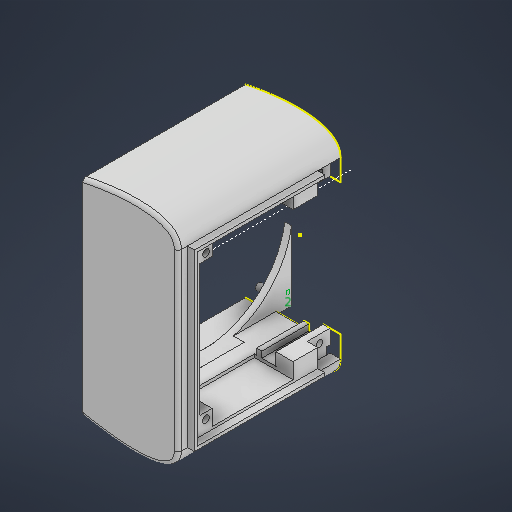
# Autodesk Inventor part: BP_FrontHSCover
Saved by Autodesk Inventor 2026.1 (Build 301233020, 233B)
## iProperties
Created: 2025-09-12
Part Number: BP_FrontHSCover
Material: Generic
Document SubType Name: Modeling
Designer: atrus
Density: 1 g/cm^3
Appearance: Default
Author: atrus
Autodesk Inventor part; units mm, degrees
ref_plane "YZ Plane" through (0, 0, 0) normal (1, 0, 0) x (0, 1, 0)
ref_plane "XZ Plane" through (0, 0, 0) normal (0, 1, 0) x (-1, 0, 0)
ref_plane "XY Plane" through (0, 0, 0) normal (0, 0, 1) x (1, 0, 0)
ref_plane "Work Plane1" through (0, 0, 0) normal (0, 0, 1) x (1, 0, 0)
sketch "Sketch1" plane through (0, 0, 0) normal (0, 0, 1) x (1, 0, 0)
  line L0 (13.335, 44.45) -> (13.335, -44.45) construction
  line L1 (5.715, 44.45) -> (13.335, 44.45) construction
  line L2 (5.715, 40.1825) -> (5.715, 44.45) construction
  arc A0 (4.9739, 39.4208) -> (5.715, 40.1825) centre (4.953, 40.1825) ccw construction
  line L3 (-12.5939, 38.9379) -> (4.9739, 39.4208) construction
  arc A1 (-12.5939, 38.9379) -> (-12.5939, 37.4145) centre (-12.573, 38.1762) ccw construction
  line L4 (4.9739, 36.9316) -> (-12.5939, 37.4145) construction
  arc A2 (5.715, 36.1699) -> (4.9739, 36.9316) centre (4.953, 36.1699) ccw construction
  line L5 (5.715, 29.2859) -> (5.715, 36.1699) construction
  arc A3 (4.9739, 28.5242) -> (5.715, 29.2859) centre (4.953, 29.2859) ccw construction
  line L6 (-12.5939, 28.0413) -> (4.9739, 28.5242) construction
  arc A4 (-12.5939, 28.0413) -> (-12.5939, 26.5179) centre (-12.573, 27.2796) ccw construction
  line L7 (4.9739, 26.035) -> (-12.5939, 26.5179) construction
  arc A5 (5.715, 25.2733) -> (4.9739, 26.035) centre (4.953, 25.2733) ccw construction
  line L8 (5.715, 18.3893) -> (5.715, 25.2733) construction
  arc A6 (4.9739, 17.6276) -> (5.715, 18.3893) centre (4.953, 18.3893) ccw construction
  line L9 (-12.5939, 17.1447) -> (4.9739, 17.6276) construction
  arc A7 (-12.5939, 17.1447) -> (-12.5939, 15.6213) centre (-12.573, 16.383) ccw construction
  line L10 (4.9739, 15.1384) -> (-12.5939, 15.6213) construction
  arc A8 (5.715, 14.3767) -> (4.9739, 15.1384) centre (4.953, 14.3767) ccw construction
  line L11 (5.715, 7.4927) -> (5.715, 14.3767) construction
  arc A9 (4.9739, 6.731) -> (5.715, 7.4927) centre (4.953, 7.4927) ccw construction
  line L12 (-12.5939, 6.2481) -> (4.9739, 6.731) construction
  arc A10 (-12.5939, 6.2481) -> (-12.5939, 4.7247) centre (-12.573, 5.4864) ccw construction
  line L13 (4.9739, 4.2418) -> (-12.5939, 4.7247) construction
  arc A11 (5.715, 3.4801) -> (4.9739, 4.2418) centre (4.953, 3.4801) ccw construction
  line L14 (5.715, -3.4039) -> (5.715, 3.4801) construction
  arc A12 (4.9739, -4.1656) -> (5.715, -3.4039) centre (4.953, -3.4039) ccw construction
  line L15 (-12.5939, -4.6485) -> (4.9739, -4.1656) construction
  arc A13 (-12.5939, -4.6485) -> (-12.5939, -6.1719) centre (-12.573, -5.4102) ccw construction
  line L16 (4.9739, -6.6548) -> (-12.5939, -6.1719) construction
  arc A14 (5.715, -7.4165) -> (4.9739, -6.6548) centre (4.953, -7.4165) ccw construction
  line L17 (5.715, -14.3005) -> (5.715, -7.4165) construction
  arc A15 (4.9739, -15.0622) -> (5.715, -14.3005) centre (4.953, -14.3005) ccw construction
  line L18 (-12.5939, -15.5451) -> (4.9739, -15.0622) construction
  arc A16 (-12.5939, -15.5451) -> (-12.5939, -17.0685) centre (-12.573, -16.3068) ccw construction
  line L19 (4.9739, -17.5514) -> (-12.5939, -17.0685) construction
  arc A17 (5.715, -18.3131) -> (4.9739, -17.5514) centre (4.953, -18.3131) ccw construction
  line L20 (5.715, -25.1971) -> (5.715, -18.3131) construction
  arc A18 (4.9739, -25.9588) -> (5.715, -25.1971) centre (4.953, -25.1971) ccw construction
  line L21 (-12.5939, -26.4417) -> (4.9739, -25.9588) construction
  arc A19 (-12.5939, -26.4417) -> (-12.5939, -27.9651) centre (-12.573, -27.2034) ccw construction
  line L22 (4.9739, -28.448) -> (-12.5939, -27.9651) construction
  arc A20 (5.715, -29.2097) -> (4.9739, -28.448) centre (4.953, -29.2097) ccw construction
  line L23 (5.715, -36.0937) -> (5.715, -29.2097) construction
  arc A21 (4.9739, -36.8554) -> (5.715, -36.0937) centre (4.953, -36.0937) ccw construction
  line L24 (-12.5939, -37.3383) -> (4.9739, -36.8554) construction
  arc A22 (-12.5939, -37.3383) -> (-12.5939, -38.8617) centre (-12.573, -38.1) ccw construction
  line L25 (4.9739, -39.3446) -> (-12.5939, -38.8617) construction
  arc A23 (5.715, -40.1063) -> (4.9739, -39.3446) centre (4.953, -40.1063) ccw construction
  line L26 (5.715, -44.45) -> (5.715, -40.1063) construction
  line L27 (13.335, -44.45) -> (5.715, -44.45) construction
  line L28 (-17.335, 44.65) -> (-17.335, 0)
  line L29 (-13.335, -62.23) -> (-13.335, 62.23) construction
  line L30 (-13.535, 0) -> (-13.535, 44.65)
  line L31 (23.335, 44.65) -> (23.335, 49.666)
  line L32 (23.335, 49.666) -> (-17.335, 49.666)
  line L33 (-17.335, 44.65) -> (-17.335, 46.4)
  line L34 (-21.835, 46) -> (-17.735, 46) construction
  line L35 (-18.8298, 48.666) -> (-20.1098, 48.666) construction
  line L36 (5.515, 44.65) -> (5.515, 41.1825)
  line L37 (5.515, 41.1825) -> (2.515, 41.1825)
  line L38 (2.515, 41.1825) -> (2.515, 44.65)
  line L39 (13.535, 44.65) -> (13.535, 37.45)
  line L40 (13.535, 37.45) -> (23.335, 37.45)
  line L41 (23.335, 37.45) -> (23.335, 44.65)
  line L42 (13.535, 44.65) -> (5.515, 44.65)
  line L43 (2.515, 44.65) -> (-13.535, 44.65)
  line L44 (-17.335, 49.666) -> (-30.735, 49.666)
  line L45 (-30.735, 49.666) -> (-30.735, 46.4)
  line L46 (-30.735, 46.4) -> (-17.335, 46.4)
  line L47 (-31.735, 46) -> (-31.735, 42) construction
  line L48 (-17.335, -62.23) -> (-17.335, 46.4) construction
  line L49 (-17.335, 49.666) -> (-17.335, 62.23) construction
  line L50 (0, 0) -> (-13.535, 0) construction
  line L51 (-17.335, -44.65) -> (-17.335, 0)
  line L52 (-13.535, 0) -> (-13.535, -44.65)
  line L53 (23.335, -44.65) -> (23.335, -49.666)
  line L54 (23.335, -49.666) -> (-17.335, -49.666)
  line L55 (-17.335, -44.65) -> (-17.335, -46.4)
  line L56 (5.515, -44.65) -> (5.515, -41.1825)
  line L57 (5.515, -41.1825) -> (2.515, -41.1825)
  line L58 (2.515, -41.1825) -> (2.515, -44.65)
  line L59 (13.535, -44.65) -> (13.535, -37.45)
  line L60 (13.535, -37.45) -> (23.335, -37.45)
  line L61 (23.335, -37.45) -> (23.335, -44.65)
  line L62 (13.535, -44.65) -> (5.515, -44.65)
  line L63 (2.515, -44.65) -> (-13.535, -44.65)
  line L64 (-17.335, -49.666) -> (-30.735, -49.666)
  line L65 (-30.735, -49.666) -> (-30.735, -46.4)
  line L66 (-30.735, -46.4) -> (-17.335, -46.4)
  line L67 (-17.335, 62.23) -> (-17.335, -46.4) construction
  point P0 (9.525, 44.45)
  point P1 (-30.735, 48.033)
  dimension "d2" = 10
  dimension "d3" = 0.2
  dimension "d4" = 1
  dimension "d5" = 1
  dimension "d6" = 0.2
  dimension "d7" = 3
  dimension "d8" = 0.2
  dimension "d10" = 0.2
  dimension "d11" = 7
  dimension "d12" = 0.4
  dimension "d13" = 1
  constraints: 74 end point, 15 symmetric about line, 10 perpendicular, 6 vertical, 4 horizontal, 4 point on line, 3 collinear, 2 midpoint, 4 other
  measures "d2" distance from line of L31.start L0
  measures "d3" distance between parallel lines of L30 L29
  measures "d4" distance between parallel lines of L32 L35
  measures "d5" distance from line of A0.centre L37
  measures "d6" distance between parallel lines of L2 L36
  measures "d7" distance of L36.end L37.end
  measures "d8" distance between parallel lines of L0 L39
  measures "d10" distance between parallel lines of L1 L42
  measures "d11" vertical distance of L0.start L39.end
  measures "d12" distance from line of L46 L34.end
  measures "d13" horizontal distance of L47.start point (-30.735, 48.033)
extrude "Extrusion1" add sketch "Sketch1" against normal blind 80
sketch "Sketch2" plane through (0, 0, -80) normal (0, 0, -1) x (-1, 0, 0)
  line L0 (17.335, -46.4) -> (17.335, 46.4) projected
  line L1 (13.535, 44.65) -> (13.535, -44.65) projected
  line L2 (13.535, 44.65) -> (13.535, 46.4)
  line L3 (13.535, 46.4) -> (17.335, 46.4)
  line L4 (13.535, -44.65) -> (-2.515, -44.65) projected
  line L5 (13.535, -44.65) -> (13.535, -46.4)
  line L6 (13.535, -46.4) -> (17.335, -46.4)
  point P0 (0, 0)
  constraints: 8 end point, 2 perpendicular, 1 point on line, 1 vertical
ref_plane "Work Plane2" through (-14.6685, -48.895, -88.9) normal (0, 0, 1) x (1, 0, 0)
extrude "Extrusion2" add sketch "Sketch2" along normal up to surface (8.9 mm away)
sketch "Sketch4" plane through (0, 0, 0) normal (0, 0, 1) x (1, 0, 0)
  line L0 (13.535, 37.45) -> (23.335, 37.45) projected
  line L1 (23.335, 37.45) -> (23.335, 49.666) projected
  line L2 (23.335, 49.666) -> (-30.735, 49.666) projected
  line L3 (-30.735, 49.666) -> (-30.735, 46.4) projected
  line L4 (-30.735, 46.4) -> (-17.335, 46.4) projected
  line L5 (-17.335, 46.4) -> (-17.335, -46.4) projected
  line L6 (-17.335, -46.4) -> (-30.735, -46.4) projected
  line L7 (-30.735, -46.4) -> (-30.735, -49.666) projected
  line L8 (-30.735, -49.666) -> (23.335, -49.666) projected
  line L9 (23.335, -49.666) -> (23.335, -37.45) projected
  line L10 (23.335, -37.45) -> (13.535, -37.45) projected
  line L11 (13.535, -37.45) -> (13.535, -44.65) projected
  line L12 (13.535, -44.65) -> (5.515, -44.65) projected
  line L13 (5.515, -44.65) -> (5.515, -41.1825) projected
  line L14 (5.515, -41.1825) -> (2.515, -41.1825) projected
  line L15 (2.515, -41.1825) -> (2.515, -44.65) projected
  line L16 (2.515, -44.65) -> (-13.535, -44.65) projected
  line L17 (-13.535, -44.65) -> (-13.535, 44.65) projected
  line L18 (-13.535, 44.65) -> (2.515, 44.65) projected
  line L19 (2.515, 44.65) -> (2.515, 41.1825) projected
  line L20 (2.515, 41.1825) -> (5.515, 41.1825) projected
  line L21 (5.515, 41.1825) -> (5.515, 44.65) projected
  line L22 (5.515, 44.65) -> (13.535, 44.65) projected
  line L23 (13.535, 44.65) -> (13.535, 37.45) projected
  point P0 (0, 0)
extrude "Extrusion3" add sketch "Sketch4" along normal blind 3.6
sketch "Sketch5" plane through (0, 0, 3.6) normal (0, 0, 1) x (1, 0, 0)
  line L0 (-30.735, 46.4) -> (-30.735, 49.666) projected
  line L1 (-30.735, -49.666) -> (23.335, -49.666) projected
  line L2 (-30.735, 49.666) -> (23.335, 49.666)
  line L3 (23.335, 49.666) -> (23.335, -49.666)
  line L4 (23.335, -49.666) -> (-30.735, -49.666)
  line L5 (-30.735, -49.666) -> (-30.735, 49.666)
  point P0 (0, 0)
  constraints: 8 end point, 2 parallel, 1 horizontal, 1 perpendicular
extrude "Extrusion4" add sketch "Sketch5" along normal blind 9
sketch "Sketch6" plane through (0, 0, 12.6) normal (0, 0, 1) x (1, 0, 0)
  line L0 (-30.735, -49.666) -> (23.335, -49.666) projected
  line L1 (23.335, 49.666) -> (-30.735, 49.666) projected
  line L2 (23.335, -49.666) -> (23.335, -63.666) construction
  line L3 (23.335, -63.666) -> (-1.735, -64.666) construction
  line L4 (23.335, -49.666) -> (-30.735, -49.666) projected
  line L5 (-1.735, -64.666) -> (-30.735, -58.666) construction
  spline S0 degree 3 poles (23.335, -49.666) (23.335, -63.666) (-1.735, -64.666) (-30.735, -58.666) knots 1 1 1 1 2 2 2 2
  line L6 (23.335, -49.666) -> (23.335, 49.666) projected
  line L7 (-14.375, 0) -> (-35.095, 0) construction
  line L8 (23.335, 49.666) -> (23.335, 63.666) construction
  line L9 (23.335, 63.666) -> (-1.735, 64.666) construction
  line L10 (-1.735, 64.666) -> (-30.735, 58.666) construction
  spline S1 degree 3 poles (23.335, 49.666) (23.335, 63.666) (-1.735, 64.666) (-30.735, 58.666) knots 1 1 1 1 2 2 2 2
  line L11 (-30.735, -49.666) -> (-30.735, -46.4) projected
  line L12 (-30.735, -49.666) -> (-30.735, -58.666)
  line L13 (-30.735, 49.666) -> (-30.735, 58.666)
  point P0 (0, 0)
  dimension "d22" = 14
  dimension "d23" = 15
  dimension "d24" = 29
  dimension "d36" = 9
  constraints: 6 end point, 2 collinear, 2 symmetric about line, 2 vertical, 1 horizontal, 8 other
  measures "d22" distance of L0.end L2.end
  measures "d23" distance from line of L0 L3.end
  measures "d24" horizontal distance of L0.start L3.end
  measures "d36" distance of L0.start L5.end
extrude "Extrusion5" add sketch "Sketch6" against normal up to surface (92.6 mm away)
sketch "Sketch18" plane through (0, 0, -80) normal (0, 0, -1) x (-1, 0, 0)
  line L0 (17.335, -46.4) -> (13.535, -46.4) projected
  line L1 (13.535, -46.4) -> (13.535, -44.65) projected
  line L2 (13.535, -44.65) -> (-2.515, -44.65) projected
  line L3 (-2.515, -44.65) -> (-2.515, -41.1825) projected
  line L4 (-2.515, -41.1825) -> (-5.515, -41.1825) projected
  line L5 (-5.515, -41.1825) -> (-5.515, -44.65) projected
  line L6 (-5.515, -44.65) -> (-13.535, -44.65) projected
  line L7 (-13.535, -44.65) -> (-13.535, -37.45) projected
  line L8 (-13.535, -37.45) -> (-23.335, -37.45) projected
  line L9 (-23.335, -37.45) -> (-23.335, -49.666) projected
  line L10 (30.735, -46.4) -> (30.735, -58.666) projected
  line L11 (30.735, -46.4) -> (17.335, -46.4) projected
  line L12 (13.535, 46.4) -> (17.335, 46.4) projected
  line L13 (17.335, 46.4) -> (30.735, 46.4) projected
  line L14 (30.735, 46.4) -> (30.735, 58.666) projected
  line L15 (-23.335, 49.666) -> (-23.335, 37.45) projected
  line L16 (-23.335, 37.45) -> (-13.535, 37.45) projected
  line L17 (-13.535, 37.45) -> (-13.535, 44.65) projected
  line L18 (-13.535, 44.65) -> (-5.515, 44.65) projected
  line L19 (-5.515, 44.65) -> (-5.515, 41.1825) projected
  line L20 (-5.515, 41.1825) -> (-2.515, 41.1825) projected
  line L21 (-2.515, 41.1825) -> (-2.515, 44.65) projected
  line L22 (-2.515, 44.65) -> (13.535, 44.65) projected
  line L23 (13.535, 44.65) -> (13.535, 46.4) projected
  point P0 (0, 0)
  constraints: 2 other
fillet "Fillet1" radius 2 3 edges at (23.335, 0, 12.6) (7.175, 61.666, 12.6) (7.175, -61.666, 12.6)
fillet "Fillet2" radius 2 2 edges at (-24.035, -46.4, 3.6) (-24.035, 46.4, 3.6)
sketch "Sketch7" plane through (0, 0, 3.6) normal (0, 0, -1) x (-1, 0, 0)
  line L0 (-13.335, 44.45) -> (-13.335, -44.45) projected
  line L1 (-5.715, 44.45) -> (-13.335, 44.45) projected
  line L2 (-5.715, 40.1825) -> (-5.715, 44.45) projected
  arc A0 (-5.715, 40.1825) -> (-4.9739, 39.4208) centre (-4.953, 40.1825) ccw projected
  line L3 (12.5939, 38.9379) -> (-4.9739, 39.4208) projected
  arc A1 (12.5939, 37.4145) -> (12.5939, 38.9379) centre (12.573, 38.1762) ccw projected
  line L4 (-4.9739, 36.9316) -> (12.5939, 37.4145) projected
  arc A2 (-4.9739, 36.9316) -> (-5.715, 36.1699) centre (-4.953, 36.1699) ccw projected
  line L5 (-5.715, 29.2859) -> (-5.715, 36.1699) projected
  arc A3 (-5.715, 29.2859) -> (-4.9739, 28.5242) centre (-4.953, 29.2859) ccw projected
  line L6 (12.5939, 28.0413) -> (-4.9739, 28.5242) projected
  arc A4 (12.5939, 26.5179) -> (12.5939, 28.0413) centre (12.573, 27.2796) ccw projected
  line L7 (-4.9739, 26.035) -> (12.5939, 26.5179) projected
  arc A5 (-4.9739, 26.035) -> (-5.715, 25.2733) centre (-4.953, 25.2733) ccw projected
  line L8 (-5.715, 18.3893) -> (-5.715, 25.2733) projected
  arc A6 (-5.715, 18.3893) -> (-4.9739, 17.6276) centre (-4.953, 18.3893) ccw projected
  line L9 (12.5939, 17.1447) -> (-4.9739, 17.6276) projected
  arc A7 (12.5939, 15.6213) -> (12.5939, 17.1447) centre (12.573, 16.383) ccw projected
  line L10 (-4.9739, 15.1384) -> (12.5939, 15.6213) projected
  arc A8 (-4.9739, 15.1384) -> (-5.715, 14.3767) centre (-4.953, 14.3767) ccw projected
  line L11 (-5.715, 7.4927) -> (-5.715, 14.3767) projected
  arc A9 (-5.715, 7.4927) -> (-4.9739, 6.731) centre (-4.953, 7.4927) ccw projected
  line L12 (12.5939, 6.2481) -> (-4.9739, 6.731) projected
  arc A10 (12.5939, 4.7247) -> (12.5939, 6.2481) centre (12.573, 5.4864) ccw projected
  line L13 (-4.9739, 4.2418) -> (12.5939, 4.7247) projected
  arc A11 (-4.9739, 4.2418) -> (-5.715, 3.4801) centre (-4.953, 3.4801) ccw projected
  line L14 (-5.715, -3.4039) -> (-5.715, 3.4801) projected
  arc A12 (-5.715, -3.4039) -> (-4.9739, -4.1656) centre (-4.953, -3.4039) ccw projected
  line L15 (12.5939, -4.6485) -> (-4.9739, -4.1656) projected
  arc A13 (12.5939, -6.1719) -> (12.5939, -4.6485) centre (12.573, -5.4102) ccw projected
  line L16 (-4.9739, -6.6548) -> (12.5939, -6.1719) projected
  arc A14 (-4.9739, -6.6548) -> (-5.715, -7.4165) centre (-4.953, -7.4165) ccw projected
  line L17 (-5.715, -14.3005) -> (-5.715, -7.4165) projected
  arc A15 (-5.715, -14.3005) -> (-4.9739, -15.0622) centre (-4.953, -14.3005) ccw projected
  line L18 (12.5939, -15.5451) -> (-4.9739, -15.0622) projected
  arc A16 (12.5939, -17.0685) -> (12.5939, -15.5451) centre (12.573, -16.3068) ccw projected
  line L19 (-4.9739, -17.5514) -> (12.5939, -17.0685) projected
  arc A17 (-4.9739, -17.5514) -> (-5.715, -18.3131) centre (-4.953, -18.3131) ccw projected
  line L20 (-5.715, -25.1971) -> (-5.715, -18.3131) projected
  arc A18 (-5.715, -25.1971) -> (-4.9739, -25.9588) centre (-4.953, -25.1971) ccw projected
  line L21 (12.5939, -26.4417) -> (-4.9739, -25.9588) projected
  arc A19 (12.5939, -27.9651) -> (12.5939, -26.4417) centre (12.573, -27.2034) ccw projected
  line L22 (-4.9739, -28.448) -> (12.5939, -27.9651) projected
  arc A20 (-4.9739, -28.448) -> (-5.715, -29.2097) centre (-4.953, -29.2097) ccw projected
  line L23 (-5.715, -36.0937) -> (-5.715, -29.2097) projected
  arc A21 (-5.715, -36.0937) -> (-4.9739, -36.8554) centre (-4.953, -36.0937) ccw projected
  line L24 (12.5939, -37.3383) -> (-4.9739, -36.8554) projected
  arc A22 (12.5939, -38.8617) -> (12.5939, -37.3383) centre (12.573, -38.1) ccw projected
  line L25 (-4.9739, -39.3446) -> (12.5939, -38.8617) projected
  arc A23 (-4.9739, -39.3446) -> (-5.715, -40.1063) centre (-4.953, -40.1063) ccw projected
  line L26 (-5.715, -44.45) -> (-5.715, -40.1063) projected
  line L27 (-13.335, -44.45) -> (-5.715, -44.45) projected
  point P0 (0, 0)
ref_plane "Work Plane3" through (-13.335, -44.45, 0) normal (0, 0, 1) x (1, 0, 0)
extrude "Extrusion6" add sketch "Sketch7" along normal up to surface (3.6 mm away)
sketch "Sketch8" plane through (-17.335, -46.4, -88.9) normal (-1, 0, 0) x (0, 0, 1)
  circle A0 centre (46, 46.4) radius 1.5 construction
  circle A1 centre (46, 46.4) radius 46.5
  line L0 (92.5, 90.8) -> (92.5, 2) projected
  point P0 (88.9, 46.4)
  point P1 (92.5, 46.4)
  constraints: 1 coincident, 1 horizontal alignment, 1 midpoint, 2 other
extrude "Extrusion7" cut sketch "Sketch8" against normal blind 10
sketch "Sketch9" plane through (-17.335, -46.4, -88.9) normal (-1, 0, 0) x (0, 0, 1)
  circle A0 centre (4.75, 5.15) radius 2.75 construction
  circle A1 centre (87.25, 5.15) radius 2.75 construction
  circle A2 centre (87.25, 87.65) radius 2.75 construction
  circle A3 centre (4.75, 87.65) radius 2.75 construction
  circle A4 centre (4.75, 87.65) radius 1.9264
  circle A5 centre (4.75, 5.15) radius 1.9264
  circle A6 centre (87.25, 5.15) radius 1.9264
  circle A7 centre (87.25, 87.65) radius 1.9264
  point P0 (88.9, 46.4)
  dimension "d33" = 3.8528
  constraints: 4 centre point, 4 coincident, 3 equal radius
  measures "d33" diameter of A5
extrude "Extrusion8" add sketch "Sketch9" along normal blind 10
sketch "Sketch10" plane through (23.335, -37.45, 3.6) normal (1, 0, 0) x (0, 0, -1)
  line L0 (83.6, 74.9) -> (0, 74.9) projected
  line L1 (83.6, 0) -> (0, 0) projected
  line L2 (56.6, 0) -> (10.5, 0)
  line L3 (10.5, 0) -> (10.5, -8.95)
  line L4 (10.5, -8.95) -> (56.6, -8.95)
  line L5 (56.6, -8.95) -> (56.6, 0)
  line L6 (0, 74.9) -> (83.6, 74.9) projected
  line L7 (56.6, 74.9) -> (10.5, 74.9)
  line L8 (10.5, 74.9) -> (10.5, 83.85)
  line L9 (10.5, 83.85) -> (56.6, 83.85)
  line L10 (56.6, 83.85) -> (56.6, 74.9)
  line L11 (0, 0) -> (0, 74.9) construction
  line L12 (128.4, 83.85) -> (174.6, 83.85) projected
  line L13 (174.6, -8.95) -> (128.4, -8.95) projected
  line L14 (83.6, 0) -> (83.6, -12.216) projected
  point P0 (10.5, -4.475)
  point P1 (56.6, -4.475)
  point P2 (10.5, 0)
  point P3 (83.6, -6.108)
  dimension "d80" = 10.5
  dimension "d81" = 27
  constraints: 16 end point, 4 collinear, 4 parallel, 3 midpoint, 2 horizontal, 2 perpendicular, 2 point on line
  measures "d80" horizontal distance of L1.end point (10.5, -4.475)
  measures "d81" horizontal distance of point (83.6, -6.108) point (56.6, -4.475)
extrude "Extrusion9" cut sketch "Sketch10" against normal blind 22
sketch "Sketch11" plane through (23.335, -49.666, -80) normal (1, 0, 0) x (0, 0, -1)
  line L0 (0, 12.216) -> (0, 0) projected
  line L1 (0, 0) -> (-90.6, 0) projected
  line L2 (0, 12.216) -> (-13, 12.216)
  line L3 (-13, 12.216) -> (-13, 0)
  line L4 (-13, 0) -> (0, 0)
  line L5 (0, 0) -> (0, 12.216)
  line L6 (-83.6, 87.116) -> (0, 87.116) projected
  line L7 (0, 87.116) -> (-13, 87.116)
  line L8 (-13, 87.116) -> (-13, 99.332)
  line L9 (-13, 99.332) -> (0, 99.332)
  line L10 (0, 99.332) -> (0, 87.116)
  line L11 (0, 99.332) -> (-90.6, 99.332) projected
  point P0 (-80, 49.666)
  point P1 (-27, 0)
  point P2 (-27, 87.116)
  point P3 (-27, 99.332)
  dimension "d42" = 13
  constraints: 16 end point, 4 parallel, 2 horizontal, 2 perpendicular, 2 point on line, 1 collinear
  measures "d42" distance between parallel lines of L0 L3
extrude "Extrusion10" cut sketch "Sketch11" against normal blind 6
sketch "Sketch12" plane through (17.335, -49.666, -80) normal (1, 0, 0) x (0, 0, -1)
  line L0 (-83.6, 87.116) -> (0, 87.116) construction
  line L1 (-5.9314, 87.116) -> (-5.9314, 98.4312) construction
  line L2 (-13, 12.216) -> (0, 12.216) construction
  point P0 (-80, 49.666)
  point P1 (-5.9314, 91.616)
  point P2 (-5.9314, 7.716)
  point P3 (-27, 87.116)
  point P4 (-6.5, 12.216)
  dimension "d45" = 4.5
  dimension "d46" = 4.5
  constraints: 2 end point, 2 point on line, 1 midpoint, 1 vertical
  measures "d45" distance from line of L0 point (-5.931, 91.616)
  measures "d46" vertical distance of point (-6.5, 12.216) point (-5.931, 7.716)
hole "Hole1" at (17.335, 41.95, -74.0686) at (17.335, -41.95, -74.0686) direction (-1, 0, 0) diameter 3.6 depth 8 tip angle 118 clearance for "Flat Head Machine Screw" size "M3" standard "Ansi Metric M Profile"
sketch "Sketch13" plane through (0, 0, -80) normal (0, 0, -1) x (-1, 0, 0)
  line L0 (-17.335, 49.666) -> (-17.335, 37.45) projected
  line L1 (-17.335, 49.666) -> (-17.335, 52.65)
  line L2 (30.735, 56.6236) -> (30.735, -56.6236) projected
  line L3 (29.735, 48.65) -> (-13.335, 48.65)
  line L4 (-13.335, 48.65) -> (-13.335, 45.65)
  line L5 (-13.335, 45.65) -> (-17.335, 45.65)
  line L6 (-17.335, 45.65) -> (-17.335, 49.666)
  line L7 (-2.515, 44.65) -> (13.535, 44.65) projected
  line L8 (0, 0) -> (53.1442, 0) construction
  line L9 (29.735, 48.65) -> (29.735, 52.65)
  line L10 (29.735, 52.65) -> (-17.335, 52.65)
  line L11 (-13.535, 44.65) -> (-5.515, 44.65) projected
  line L12 (-17.335, 47.658) -> (-17.335, 45.65)
  line L13 (-17.335, -49.666) -> (-17.335, -52.65)
  line L14 (29.735, -48.65) -> (-13.335, -48.65)
  line L15 (-13.335, -48.65) -> (-13.335, -45.65)
  line L16 (-13.335, -45.65) -> (-17.335, -45.65)
  line L17 (-17.335, -45.65) -> (-17.335, -49.666)
  line L18 (29.735, -48.65) -> (29.735, -52.65)
  line L19 (29.735, -52.65) -> (-17.335, -52.65)
  point P0 (30.735, 53.6088)
  point P1 (-13.335, 47.15)
  point P2 (-15.335, 45.65)
  point P3 (5.51, 44.65)
  point P4 (30.735, 48.65)
  dimension "d55" = 4
  dimension "d57" = 4
  dimension "d60" = 4
  dimension "d61" = 1
  dimension "d62" = 1
  constraints: 32 end point, 7 symmetric about line, 4 midpoint, 3 horizontal, 3 point on line, 2 perpendicular, 1 parallel, 1 vertical
  measures "d55" horizontal distance of L12.start point (-13.335, 47.15)
  measures "d57" distance from line of point (5.51, 44.65) L3
  measures "d60" distance of L3.start L9.end
  measures "d61" distance between parallel lines of L2 L9
  measures "d62" distance between parallel lines of L11 L5
extrude "Extrusion11" cut sketch "Sketch13" against normal blind 2
sketch "Sketch14" plane through (-30.735, 46.4, -80) normal (-1, 0, 0) x (0, 0, 1)
  arc A0 (81.6, -92.8) -> (83.6, -90.8) centre (81.6, -90.8) ccw construction
  arc A1 (83.6, -2) -> (81.6, 0) centre (81.6, -2) ccw construction
  line L0 (90.6, 12.266) -> (0, 12.266) construction
  line L1 (90.6, -105.066) -> (0, -105.066) construction
  line L2 (0, -92.8) -> (81.6, -92.8) construction
  line L3 (-4.9, -0.4) -> (79.1, -0.4) construction
  line L4 (0, -98.933) -> (56.2544, -98.933) construction
  line L5 (0, 3.266) -> (0, 6.25) construction
  line L6 (0, 4.758) -> (15.1017, 4.758) construction
  line L7 (90.6, -105.066) -> (92.5996, -103.0648) construction
  line L8 (91.5998, -104.0654) -> (83.0142, -92.2142) construction
  line L9 (90.6, 12.266) -> (90.6, 12.266) construction
  line L10 (83.0142, -0.5858) -> (90.6, 12.266) construction
  line L11 (8, 12.266) -> (8, -105.066) construction
  line L12 (0, 0) -> (0, 12.266) construction
  circle A2 centre (8, -98.933) radius 2
  circle A3 centre (8, 4.758) radius 2
  circle A4 centre (87.307, -98.1398) radius 2
  circle A5 centre (86.8071, 5.8401) radius 2
  line L13 (0, -92.8) -> (0, -105.066) projected
  point P0 (80, -46.4)
  point P1 (0, 6.133)
  dimension "d63" = 8
  dimension "d64" = 4
  constraints: 14 end point, 7 midpoint, 6 coincident, 6 point on line, 4 centre point, 3 equal radius, 2 horizontal, 2 point on circle, 1 perpendicular, 4 other
  measures "d63" distance from line of point (0, 6.133) L11
  measures "d64" diameter of A5
extrude "Extrusion12" cut sketch "Sketch14" against normal blind 7
sketch "Sketch15" plane through (0, 0, 3.6) normal (0, 0, -1) x (-1, 0, 0)
  line L0 (-23.335, -37.45) -> (-23.335, 37.45) projected
  line L1 (-23.335, -37.45) -> (-13.535, -37.45) projected
  line L2 (-23.335, 37.45) -> (-13.535, 37.45)
  line L3 (-13.535, 37.45) -> (-13.535, -37.45)
  line L4 (-13.535, -37.45) -> (-23.335, -37.45)
  line L5 (-23.335, -37.45) -> (-23.335, 37.45)
  line L6 (-13.335, -44.45) -> (-13.335, 44.45) projected
  point P0 (0, 0)
  dimension "d69" = 0.2
  constraints: 8 end point, 2 parallel, 1 horizontal, 1 perpendicular, 1 point on line
  measures "d69" distance between parallel lines of L6 L3
extrude "Extrusion13" add sketch "Sketch15" along normal blind 3.5
sketch "Sketch16" plane through (-17.335, -46.4, -88.9) normal (-1, 0, 0) x (0, 0, 1)
  line L0 (8.9, 0) -> (0, 0) projected
  line L1 (0, 0) -> (8.9, 0)
  line L2 (8.9, 0) -> (8.9, 2)
  line L3 (8.9, 2) -> (0, 2)
  line L4 (0, 2) -> (0, 0)
  line L5 (92.5, 90.8) -> (92.5, 2) projected
  line L6 (92.5, 46.4) -> (-38.4261, 46.4) construction
  line L7 (8.9, 92.8) -> (0, 92.8)
  line L8 (0, 92.8) -> (8.9, 92.8)
  line L9 (8.9, 92.8) -> (8.9, 90.8)
  line L10 (8.9, 90.8) -> (0, 90.8)
  line L11 (0, 90.8) -> (0, 92.8)
  point P0 (88.9, 46.4)
  dimension "d72" = 2
  constraints: 20 end point, 5 symmetric about line, 2 horizontal, 2 parallel, 1 midpoint, 1 perpendicular
  measures "d72" distance of L3.end L0.end
sketch "Sketch17" plane through (23.335, -49.666, 10.6) normal (1, 0, 0) x (0, 0, -1)
  line L0 (0, 0) -> (0, 99.332) projected
  line L1 (77.6, 99.332) -> (0, 99.332) projected
  line L2 (77.6, 0) -> (0, 0) projected
  line L3 (77.6, 87.116) -> (77.6, 99.332) projected
  line L4 (77.6, 97.532) -> (5.2, 97.532)
  line L5 (5.2, 97.532) -> (5.2, 1.8)
  line L6 (5.2, 1.8) -> (77.6, 1.8)
  line L7 (77.6, 0) -> (77.6, 12.216) projected
  line L8 (3.4, 0) -> (3.4, 99.332)
  point P0 (10.6, 49.666)
  dimension "d74" = 1.8
  dimension "d75" = 5.2
  dimension "d76" = 1.8
  dimension "d86" = 1.8
  constraints: 8 end point, 3 point on line, 2 parallel, 1 horizontal, 1 perpendicular
  measures "d74" distance between parallel lines of L2 L6
  measures "d75" distance between parallel lines of L0 L5
  measures "d76" distance between parallel lines of L4 L1
  measures "d86" distance between parallel lines of L5 L8
extrude "Cover Glass Frame" add sketch "Sketch17" along normal blind 4 contours L8 L1 L3 L4 L5 L6 L7 L2
sketch "Sketch19" plane through (23.335, -46.4, -53) normal (1, 0, 0) x (0, 0, -1)
  circle A0 centre (-49.6, 87.35) radius 1.2295 projected
  circle A1 centre (-49.6, 5.45) radius 1.2295 projected
  circle A2 centre (-49.6, 87.35) radius 1.9
  circle A3 centre (-49.6, 5.45) radius 1.9
  point P0 (-53, 46.4)
  dimension "d82" = 3.8
  dimension "d83" = 3.8
  constraints: 2 centre point, 2 coincident
  measures "d82" diameter of A2
  measures "d83" diameter of A3
extrude "Extrusion15" cut sketch "Sketch19" against normal blind 10 contours A0 | A1 | A2 | A3
body "Solid1"
